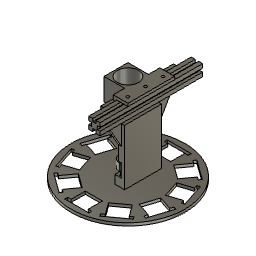
27.10_Derzhatel_motor_turel (Autodesk Fusion 360 design; units mm, degrees)
Autodesk Fusion 360 part; units mm, degrees
note: some values were not read from the file. Set by a fixed rule: which sketch regions a step uses.
sketch "Sketch1" plane through (0, 0, 0) normal (0, 0, 1) x (1, 0, 0)
  circle A0 centre (0, 0) radius 4
  dimension "d1" = 8
  constraint coincident A0.centre origin
  measures "d1" diameter of A0
sketch "Sketch2" plane through (0, 0, 0) normal (0, 0, 1) x (1, 0, 0)
  line L0 (-21, 21) -> (21, 21)
  line L1 (21, 21) -> (21, -21)
  line L2 (21, -21) -> (-21, -21)
  line L3 (-21, -21) -> (-21, 21)
  line L4 (-21, 21) -> (21, -21) construction
  circle A0 centre (0, 0) radius 4
  dimension "d4" = 42
  constraint horizontal L0
  constraint vertical L1
  constraint horizontal L2
  constraint vertical L3
  constraint equal L0 L3
  constraint midpoint A0.centre L4
  measures "d4" distance of L0.start L0.end
extrude "Extrude2" add sketch "Sketch2" along normal blind 8 makes body 1
sketch "Sketch3" plane through (0, 0, 8) normal (0, 0, 1) x (-1, 0, 0)
  circle A0 centre (0, 0) radius 4
  line L0 (21, 21) -> (-21, 21)
  line L1 (-21, 21) -> (-21, -21)
  line L2 (-21, -21) -> (21, -21)
  line L3 (21, -21) -> (21, 21)
  circle A1 centre (0, 0) radius 11.1
  line L4 (-10, 10) -> (10, 10)
  line L5 (10, 10) -> (10, -10)
  line L6 (10, -10) -> (-10, -10)
  line L7 (-10, -10) -> (-10, 10)
  line L8 (-10, 10) -> (10, -10) construction
  circle A2 centre (10, 10) radius 1.25
  circle A3 centre (10, -10) radius 1.25
  circle A4 centre (-10, 10) radius 1.25
  circle A5 centre (-10, -10) radius 1.25
  circle A6 centre (0, 0) radius 18.5
  dimension "d7" = 22.2
  dimension "d8" = 20
  dimension "d9" = 2.5
  dimension "d10" = 2.5
  dimension "d11" = 2.5
  dimension "d12" = 2.5
  dimension "d16" = 37
  constraint coincident A0.centre A1.centre
  constraint horizontal L4
  constraint vertical L5
  constraint horizontal L6
  constraint vertical L7
  constraint equal L4 L7
  constraint midpoint A0.centre L8
  constraint coincident L4.end L5.start
  constraint coincident L5.end L6.start
  constraint coincident L4.start L7.end
  constraint coincident L6.end L7.start
  measures "d7" diameter of A1
  measures "d8" distance of L4.start L4.end
  measures "d9" diameter of A2
  measures "d10" diameter of A3
  measures "d11" diameter of A4
  measures "d12" diameter of A5
  measures "d16" diameter of A6
extrude "Extrude3" cut sketch "Sketch3" against normal through all contours L4 L5 A2 | L4 L5 A2 | L5 L6 A3 | L5 L6 A3 | L4 L7 A4 | L4 L7 A4 | L6 L7 A5 | L6 L7 A5 bodies 1
extrude "Extrude4" cut sketch "Sketch3" against normal blind 2 contours A1 L5 | A1 L4 L5 L6 L7 | A1 L4 | A1 L6 | A1 L7 bodies 1
extrude "Extrude5" add sketch "Sketch3" along normal blind 31 contours L0 L1 L2 L3 bodies 1
sketch "Sketch4" plane through (21, 0, 0) normal (1, 0, 0) x (0, 1, 0)
  line L0 (-21, 0) -> (21, 0)
  line L1 (21, 0) -> (21, 39)
  line L2 (21, 39) -> (-21, 39)
  line L3 (-21, 39) -> (-21, 0)
  line L4 (-41, 39) -> (41, 39)
  line L5 (41, 39) -> (41, 14)
  line L6 (41, 14) -> (-41, 14)
  line L7 (-41, 14) -> (-41, 39)
  line L8 (-41, 39) -> (41, 39)
  line L9 (41, 39) -> (41, 34)
  line L10 (41, 34) -> (-41, 34)
  line L11 (-41, 34) -> (-41, 39)
  line L12 (21, 34) -> (41, 14) construction
  line L13 (41, 34) -> (21, 14) construction
  line L14 (41, 24.1296) -> (-41, 24.1296) construction
  circle A0 centre (31, 24) radius 2.5
  circle A1 centre (-31.4227, 24.1296) radius 2.5
  dimension "d19" = 25
  dimension "d20" = 20
  dimension "d21" = 20
  dimension "d24" = 5
  dimension "d27" = 5
  dimension "d28" = 5
  constraint horizontal L4
  constraint vertical L5
  constraint horizontal L6
  constraint vertical L7
  constraint horizontal L8
  constraint vertical L9
  constraint horizontal L10
  constraint vertical L11
  constraint coincident L1 L12.start
  constraint coincident L10 L12.start
  constraint coincident L6 L13.end
  constraint coincident L1 L13.end
  constraint coincident L5 L14.start
  constraint coincident L7 L14.end
  constraint perpendicular L7 L14
  constraint midpoint L13 A0.centre
  constraint coincident L14 A1.centre
  measures "d19" distance of L4.start L6.end
  measures "d20" distance of L3 L7
  measures "d21" distance of L1 L5
  measures "d24" distance of L4.start L10.end
  measures "d27" diameter of A0
  measures "d28" diameter of A1
extrude "Extrude6" add sketch "Sketch4" against normal blind 6 contours L3 L6 L7 L10 | L1 L5 L6 L10 | L3 L4 L7 L8 L10 L11 | L1 L4 L5 L8 L9 L10 | A0 | A1 bodies 1
extrude "Extrude7" add sketch "Sketch4" along normal blind 20 contours L3 L4 L7 L8 L10 L11 | L1 L2 L3 L4 L8 L10 | L1 L4 L5 L8 L9 L10 bodies 1
extrude "Extrude8" cut sketch "Sketch4" against normal through all contours A0 | A1 bodies 1
sketch "Sketch5" plane through (0, 0, 34) normal (0, 0, -1) x (1, 0, 0)
  line L0 (21, 41) -> (21, -41)
  line L1 (21, -41) -> (41, -41)
  line L2 (41, -41) -> (41, 41)
  line L3 (41, 41) -> (21, 41)
  line L4 (21, -41) -> (41, 41) construction
  line L5 (21, 41) -> (41, -41) construction
  line L6 (31, 41) -> (31, -41) construction
  circle A0 centre (31, 31.2813) radius 2.5
  circle A1 centre (31, 0) radius 2.5
  circle A2 centre (31, -30.6847) radius 2.5
  dimension "d30" = 5
  dimension "d31" = 5
  dimension "d32" = 5
  constraint coincident L0.end L1.start
  constraint coincident L2.end L3.start
  constraint coincident L0.start L3.end
  constraint coincident L1.end L2.start
  constraint midpoint L3 L6.start
  constraint perpendicular L3 L6
  constraint coincident L6 A0.centre
  constraint midpoint L5 A1.centre
  constraint coincident L6 A2.centre
  measures "d30" diameter of A0
  measures "d31" diameter of A1
  measures "d32" diameter of A2
extrude "Extrude9" cut sketch "Sketch5" against normal through all contours A0 | A1 | A2 bodies 1
ref_plane "WorkPlane1" through (0, 0, -2) normal (0, 0, -1) x (-1, 0, 0)
sketch "Sketch7" plane through (0, 0, -2) normal (0, 0, -1) x (1, 0, 0)
  circle A0 centre (0, 0) radius 4
  circle A1 centre (0, 0) radius 9.5
  dimension "d35" = 8
  dimension "d36" = 19
  constraint coincident A0.centre A1.centre
  measures "d35" diameter of A0
  measures "d36" diameter of A1
extrude "Extrude10" add sketch "Sketch7" along normal blind 19 separate body contours A0 | A1 makes body 2
sketch "Sketch10" plane through (0, 0, -21) normal (0, 0, -1) x (1, 0, 0)
  circle A0 centre (0, 0) radius 9.5
  circle A1 centre (0, 0) radius 4
extrude "Extrude13" add sketch "Sketch10" along normal blind 35 contours A1 bodies 2
sketch "Sketch11" plane through (0, 0, -56) normal (0, 0, -1) x (1, 0, 0)
  circle A0 centre (0, 0) radius 4
  line L0 (-6.5, -3.7528) -> (0, -7.5056)
  line L1 (0, -7.5056) -> (6.5, -3.7528)
  line L2 (6.5, -3.7528) -> (6.5, 3.7528)
  line L3 (6.5, 3.7528) -> (0, 7.5056)
  line L4 (0, 7.5056) -> (-6.5, 3.7528)
  line L5 (-6.5, 3.7528) -> (-6.5, -3.7528)
  dimension "d48" = 13
  constraint coincident A0.centre origin
  constraint vertical L5
  measures "d48" distance of L2 L5
extrude "Extrude14" add sketch "Sketch11" along normal blind 5 contours A0 | L0 L1 L2 L3 L4 L5 bodies 2
extrude "Extrude15" add sketch "Sketch7" against normal blind 10 contours A0 bodies 2
ref_plane "WorkPlane2" through (0, 0, -63) normal (0, 0, -1) x (-1, 0, 0)
sketch "Sketch12" plane through (0, 0, -63) normal (0, 0, -1) x (1, 0, 0)
  line L0 (-6.5, 3.7528) -> (-6.5, -3.7528)
  line L1 (-6.5, -3.7528) -> (0, -7.5056)
  line L2 (0, -7.5056) -> (6.5, -3.7528)
  line L3 (6.5, -3.7528) -> (6.5, 3.7528)
  line L4 (6.5, 3.7528) -> (0, 7.5056)
  line L5 (0, 7.5056) -> (-6.5, 3.7528)
extrude "Extrude16" add sketch "Sketch12" along normal blind 5 separate body makes body 3
sketch "Sketch13" plane through (0, 0, -68) normal (0, 0, -1) x (1, 0, 0)
  line L0 (0, 7.5056) -> (-6.5, 3.7528)
  line L1 (-6.5, 3.7528) -> (-6.5, -3.7528)
  line L2 (-6.5, -3.7528) -> (0, -7.5056)
  line L3 (0, -7.5056) -> (6.5, -3.7528)
  line L4 (6.5, -3.7528) -> (6.5, 3.7528)
  line L5 (6.5, 3.7528) -> (0, 7.5056)
  circle A0 centre (0, 0) radius 4
extrude "Extrude17" add sketch "Sketch13" along normal blind 45 contours A0 bodies 3
sketch "Sketch14" plane through (0, 0, -113) normal (0, 0, -1) x (1, 0, 0)
  circle A0 centre (0, 0) radius 4
  circle A1 centre (0, 0) radius 100
  line L0 (-21, -90) -> (21, -90)
  line L1 (21, -90) -> (21, -85)
  line L2 (21, -85) -> (15, -85)
  line L3 (15, -85) -> (15, -60)
  line L4 (15, -60) -> (-15, -60)
  line L5 (-15, -60) -> (-15, -85)
  line L6 (-15, -85) -> (-21, -85)
  line L7 (-21, -85) -> (-21, -90)
  line L8 (0, -60) -> (0, -90) construction
  line L9 (62.097, -59.9497) -> (47.4024, -39.7242)
  line L10 (47.4024, -39.7242) -> (23.1319, -57.3578)
  line L11 (23.1319, -57.3578) -> (37.8265, -77.5832)
  line L12 (37.8265, -77.5832) -> (32.9724, -81.1099)
  line L13 (32.9724, -81.1099) -> (35.9113, -85.155)
  line L14 (35.9113, -85.155) -> (69.89, -60.468)
  line L15 (69.89, -60.468) -> (66.9511, -56.423)
  line L16 (66.9511, -56.423) -> (62.097, -59.9497)
  line L17 (85.4751, -12.0006) -> (61.6986, -4.2752)
  line L18 (61.6986, -4.2752) -> (52.4281, -32.8069)
  line L19 (52.4281, -32.8069) -> (76.2045, -40.5323)
  line L20 (76.2045, -40.5323) -> (74.3504, -46.2386)
  line L21 (74.3504, -46.2386) -> (79.1057, -47.7837)
  line L22 (79.1057, -47.7837) -> (92.0844, -7.8393)
  line L23 (92.0844, -7.8393) -> (87.3292, -6.2943)
  line L24 (87.3292, -6.2943) -> (85.4751, -12.0006)
  line L25 (76.2045, 40.5323) -> (52.4281, 32.8069)
  line L26 (52.4281, 32.8069) -> (61.6986, 4.2752)
  line L27 (61.6986, 4.2752) -> (85.4751, 12.0006)
  line L28 (85.4751, 12.0006) -> (87.3292, 6.2943)
  line L29 (87.3292, 6.2943) -> (92.0844, 7.8393)
  line L30 (92.0844, 7.8393) -> (79.1057, 47.7837)
  line L31 (79.1057, 47.7837) -> (74.3504, 46.2386)
  line L32 (74.3504, 46.2386) -> (76.2045, 40.5323)
  line L33 (37.8265, 77.5832) -> (23.1319, 57.3578)
  line L34 (23.1319, 57.3578) -> (47.4024, 39.7242)
  line L35 (47.4024, 39.7242) -> (62.097, 59.9497)
  line L36 (62.097, 59.9497) -> (66.9511, 56.423)
  line L37 (66.9511, 56.423) -> (69.89, 60.468)
  line L38 (69.89, 60.468) -> (35.9113, 85.155)
  line L39 (35.9113, 85.155) -> (32.9724, 81.1099)
  line L40 (32.9724, 81.1099) -> (37.8265, 77.5832)
  line L41 (-15, 85) -> (-15, 60)
  line L42 (-15, 60) -> (15, 60)
  line L43 (15, 60) -> (15, 85)
  line L44 (15, 85) -> (21, 85)
  line L45 (21, 85) -> (21, 90)
  line L46 (21, 90) -> (-21, 90)
  line L47 (-21, 90) -> (-21, 85)
  line L48 (-21, 85) -> (-15, 85)
  line L49 (-62.097, 59.9497) -> (-47.4024, 39.7242)
  line L50 (-47.4024, 39.7242) -> (-23.1319, 57.3578)
  line L51 (-23.1319, 57.3578) -> (-37.8265, 77.5832)
  line L52 (-37.8265, 77.5832) -> (-32.9724, 81.1099)
  line L53 (-32.9724, 81.1099) -> (-35.9113, 85.155)
  line L54 (-35.9113, 85.155) -> (-69.89, 60.468)
  line L55 (-69.89, 60.468) -> (-66.9511, 56.423)
  line L56 (-66.9511, 56.423) -> (-62.097, 59.9497)
  line L57 (-85.4751, 12.0006) -> (-61.6986, 4.2752)
  line L58 (-61.6986, 4.2752) -> (-52.4281, 32.8069)
  line L59 (-52.4281, 32.8069) -> (-76.2045, 40.5323)
  line L60 (-76.2045, 40.5323) -> (-74.3504, 46.2386)
  line L61 (-74.3504, 46.2386) -> (-79.1057, 47.7837)
  line L62 (-79.1057, 47.7837) -> (-92.0844, 7.8393)
  line L63 (-92.0844, 7.8393) -> (-87.3292, 6.2943)
  line L64 (-87.3292, 6.2943) -> (-85.4751, 12.0006)
  line L65 (-76.2045, -40.5323) -> (-52.4281, -32.8069)
  line L66 (-52.4281, -32.8069) -> (-61.6986, -4.2752)
  line L67 (-61.6986, -4.2752) -> (-85.4751, -12.0006)
  line L68 (-85.4751, -12.0006) -> (-87.3292, -6.2943)
  line L69 (-87.3292, -6.2943) -> (-92.0844, -7.8393)
  line L70 (-92.0844, -7.8393) -> (-79.1057, -47.7837)
  line L71 (-79.1057, -47.7837) -> (-74.3504, -46.2386)
  line L72 (-74.3504, -46.2386) -> (-76.2045, -40.5323)
  line L73 (-37.8265, -77.5832) -> (-23.1319, -57.3578)
  line L74 (-23.1319, -57.3578) -> (-47.4024, -39.7242)
  line L75 (-47.4024, -39.7242) -> (-62.097, -59.9497)
  line L76 (-62.097, -59.9497) -> (-66.9511, -56.423)
  line L77 (-66.9511, -56.423) -> (-69.89, -60.468)
  line L78 (-69.89, -60.468) -> (-35.9113, -85.155)
  line L79 (-35.9113, -85.155) -> (-32.9724, -81.1099)
  line L80 (-32.9724, -81.1099) -> (-37.8265, -77.5832)
  dimension "d58" = 200
  dimension "d59" = 60
  dimension "d60" = 30
  dimension "d61" = 5
  dimension "d62" = 42
  dimension "d63" = 30
  dimension "d65" = 360
  constraint coincident A0.centre A1.centre
  constraint horizontal L0
  constraint perpendicular L0 L1
  constraint perpendicular L1 L2
  constraint perpendicular L2 L3
  constraint perpendicular L1 L4
  constraint perpendicular L4 L5
  constraint perpendicular L1 L6
  constraint perpendicular L0 L7
  constraint equal L2 L6
  constraint midpoint L4 L8.start
  constraint midpoint L0 L8.end
  constraint coincident A0.centre L8
  constraint equal L1 L7
  measures "d58" diameter of A1
  measures "d59" distance of A0.centre L4
  measures "d60" distance of L0 L4
  measures "d61" distance of L0.end L1.end
  measures "d62" distance of L0.start L0.end
  measures "d63" distance of L3.end L4.end
extrude "Extrude18" add sketch "Sketch14" along normal blind 5 contours A0 | A1 bodies 3
ref_plane "WorkPlane3" through (0, 0, -99) normal (0, 0, 1) x (-1, 0, 0)
sketch "Sketch15" plane through (0, 0, -99) normal (0, 0, 1) x (1, 0, 0)
  circle A0 centre (0, 0) radius 14.5
  line L0 (14.5, -27.5) -> (14.5, 27.5)
  line L1 (14.5, 27.5) -> (19.5, 27.5)
  line L2 (19.5, 27.5) -> (19.5, -27.5)
  line L3 (19.5, -27.5) -> (14.5, -27.5)
  circle A1 centre (0, 0) radius 4
  line L4 (19.5, 0) -> (14.5, 0) construction
  line L5 (0, -14.5) -> (14.5, -14.5)
  line L6 (0, 14.5) -> (14.5, 14.5)
  dimension "d69" = 29
  dimension "d74" = 8
  dimension "d77" = 5
  dimension "d78" = 55
  constraint coincident A0.centre A1.centre
  constraint concentric A0 A1
  constraint tangent A0 L0
  constraint vertical L0
  constraint vertical L2
  constraint horizontal L3
  constraint horizontal L1
  constraint midpoint L2 L4.start
  constraint midpoint L0 L4.end
  constraint coincident A0.centre L4
  constraint coincident A0 L5.start
  constraint coincident L0 L5.end
  constraint tangent A0 L5
  constraint coincident A0 L6.start
  constraint coincident L0 L6.end
  constraint tangent A0 L6
  constraint horizontal L5
  constraint horizontal L6
  measures "d69" diameter of A0
  measures "d74" diameter of A1
  measures "d77" distance of L0.start L2.end
  measures "d78" distance of L1.end L2.end
extrude "Extrude20" add sketch "Sketch15" along normal blind 13 bodies 3
sketch "Sketch16" plane through (0, 0, 0) normal (0, 1, 0) x (1, 0, 0)
  line L0 (21, -34) -> (41, -34)
  line L1 (21, -34) -> (21, -14)
  line L2 (21, -34) -> (41, -34)
  line L3 (21, -34) -> (21, -14)
  line L4 (21, -14) -> (41, -14)
  line L5 (41, -14) -> (41, -34)
  line L6 (31, -34) -> (31, -14) construction
  line L7 (41, -24) -> (21, -24) construction
  line L8 (21, -24) -> (21, -27)
  line L9 (21, -27) -> (26, -27)
  line L10 (26, -27) -> (26, -21)
  line L11 (26, -21) -> (21, -21)
  circle A0 centre (31, -24) radius 1.5 construction
  line L12 (28, -29) -> (28, -34)
  line L13 (34, -29) -> (28, -29)
  line L14 (34, -34) -> (34, -29)
  line L15 (36, -27) -> (41, -27)
  line L16 (36, -21) -> (36, -27)
  line L17 (41, -21) -> (36, -21)
  line L18 (34, -19) -> (34, -14)
  line L19 (28, -19) -> (34, -19)
  line L20 (28, -14) -> (28, -19)
  dimension "d81" = 3
  dimension "d82" = 6
  dimension "d83" = 5
  dimension "d84" = 3
  dimension "d86" = 360
  constraint coincident L0.start L1.start
  constraint coincident L0.end L2.end
  constraint coincident L1.end L3.end
  constraint perpendicular L3 L4
  constraint perpendicular L0 L5
  constraint midpoint L0 L6.start
  constraint midpoint L4 L6.end
  constraint midpoint L5 L7.start
  constraint midpoint L3 L7.end
  constraint perpendicular L7 L8
  constraint perpendicular L3 L9
  constraint perpendicular L7 L10
  constraint coincident L3 L11.end
  constraint perpendicular L3 L11
  constraint midpoint L7 A0.centre
  measures "d81" distance of L7.end L8.end
  measures "d82" distance of L9.end L10.end
  measures "d83" distance of L8.end L9.end
  measures "d84" diameter of A0
extrude "Extrude21" add sketch "Sketch16" along normal mid plane 180 separate body contours L0 L1 L2 L3 L4 L5 L9 L10 L11 L12 L13 L14 L15 L16 L17 L18 L19 L20 makes body 4
ref_plane "WorkPlane4" through (20.5, 0, -92.5) normal (1, 0, 0) x (0, 1, 0)
sketch "Sketch17" plane through (20.5, 0, -92.5) normal (1, 0, 0) x (0, 1, 0)
  line L0 (27.5, -6.5) -> (-27.5, -6.5)
  line L1 (-27.5, -6.5) -> (27.5, -6.5)
  line L2 (27.5, -6.5) -> (27.5, 6.5)
  line L3 (27.5, 6.5) -> (-27.5, 6.5)
  line L4 (-27.5, 6.5) -> (-27.5, -6.5)
  line L5 (-32.5, 6.5) -> (32.5, 6.5)
  line L6 (32.5, 6.5) -> (32.5, -11.5)
  line L7 (32.5, -11.5) -> (-32.5, -11.5)
  line L8 (-32.5, -11.5) -> (-32.5, 6.5)
  dimension "d88" = 5
  dimension "d89" = 5
  dimension "d90" = 5
  constraint horizontal L5
  constraint vertical L6
  constraint horizontal L7
  constraint vertical L8
  constraint collinear L3 L5
  measures "d88" distance of L2 L6
  measures "d89" distance of L4 L8
  measures "d90" distance of L0 L7
extrude "Extrude22" add sketch "Sketch17" along normal blind 6 separate body makes body 5
sketch "Sketch18" plane through (20.5, 0, 0) normal (-1, 0, 0) x (0, -1, 0)
  line L0 (-32.5, -104) -> (32.5, -104)
  line L1 (32.5, -104) -> (32.5, -86)
  line L2 (32.5, -86) -> (-32.5, -86)
  line L3 (-32.5, -86) -> (-32.5, -104)
  line L4 (27.5, -99) -> (14.5, -99)
  line L5 (-14.5, -99) -> (-27.5, -99)
  line L6 (-27.5, -99) -> (-14.5, -99)
  line L7 (-14.5, -99) -> (-14.5, -86)
  line L8 (-14.5, -86) -> (-27.5, -86)
  line L9 (-27.5, -86) -> (-27.5, -99)
  line L10 (14.5, -99) -> (27.5, -99)
  line L11 (27.5, -99) -> (27.5, -86)
  line L12 (27.5, -86) -> (14.5, -86)
  line L13 (14.5, -86) -> (14.5, -99)
  line L14 (32.5, -104) -> (21, -104)
  line L15 (21, -104) -> (21, -99)
  line L16 (21, -99) -> (32.5, -99)
  line L17 (32.5, -99) -> (32.5, -104)
  line L18 (-32.5, -104) -> (-21, -104)
  line L19 (-21, -104) -> (-21, -99)
  line L20 (-21, -99) -> (-32.5, -99)
  line L21 (-32.5, -99) -> (-32.5, -104)
  line L22 (-21, -104) -> (21, -104)
  line L23 (21, -104) -> (21, -99)
  line L24 (21, -99) -> (-21, -99)
  line L25 (-21, -99) -> (-21, -104)
  constraint horizontal L14
  constraint vertical L15
  constraint horizontal L16
  constraint vertical L17
  constraint midpoint L10 L15.end
  constraint coincident L0.end L1.start
  constraint horizontal L18
  constraint vertical L19
  constraint horizontal L20
  constraint vertical L21
  constraint midpoint L6 L19.end
  constraint coincident L0.start L3.end
  constraint horizontal L22
  constraint vertical L23
  constraint horizontal L24
  constraint vertical L25
extrude "Extrude23" add sketch "Sketch18" along normal blind 11 contours L0 L3 L5 L6 L18 L19 L20 L21 L25 | L0 L4 L5 L6 L10 L15 L19 L22 L23 L24 L25 | L0 L1 L4 L10 L14 L15 L16 L17 L23 bodies 5
sketch "Sketch19" plane through (0, 0, -99) normal (0, 0, 1) x (-1, 0, 0)
  line L0 (-9.5, -32.5) -> (-9.5, 32.5)
  line L1 (-9.5, 32.5) -> (-20.5, 32.5)
  line L2 (-20.5, 32.5) -> (-20.5, -32.5)
  line L3 (-20.5, -32.5) -> (-9.5, -32.5)
  circle A0 centre (0, 0) radius 4
  arc A1 (0, -14.5) -> (0, 14.5) centre (0, 0) ccw
  line L4 (0, 14.5) -> (-14.5, 14.5)
  line L5 (-14.5, 14.5) -> (-14.5, 27.5)
  line L6 (-14.5, 27.5) -> (-19.5, 27.5)
  line L7 (-19.5, 27.5) -> (-19.5, -27.5)
  line L8 (-19.5, -27.5) -> (-14.5, -27.5)
  line L9 (-14.5, -27.5) -> (-14.5, -14.5)
  line L10 (-14.5, -14.5) -> (0, -14.5)
  line L11 (-9.5, 32.5) -> (-14.5, 32.5)
  line L12 (-14.5, 32.5) -> (-14.5, 18.5)
  line L13 (-14.5, 18.5) -> (-9.5, 18.5)
  line L14 (-9.5, 18.5) -> (-9.5, 32.5)
  line L15 (-9.5, -32.5) -> (-14.5, -32.5)
  line L16 (-14.5, -32.5) -> (-14.5, -18.5)
  line L17 (-14.5, -18.5) -> (-9.5, -18.5)
  line L18 (-9.5, -18.5) -> (-9.5, -32.5)
  line L19 (-14.5, -32.5) -> (-20.5, -32.5)
  line L20 (-20.5, -32.5) -> (-20.5, -29.5)
  line L21 (-20.5, -29.5) -> (-14.5, -29.5)
  line L22 (-14.5, -29.5) -> (-14.5, -32.5)
  line L23 (-14.5, 32.5) -> (-20.5, 32.5)
  line L24 (-20.5, 32.5) -> (-20.5, 29.5)
  line L25 (-20.5, 29.5) -> (-14.5, 29.5)
  line L26 (-14.5, 29.5) -> (-14.5, 32.5)
  dimension "d95" = 14
  dimension "d99" = 2
  constraint horizontal L11
  constraint vertical L12
  constraint horizontal L13
  constraint vertical L14
  constraint coincident L5 L12.end
  constraint coincident L0.end L1.start
  constraint horizontal L15
  constraint vertical L16
  constraint horizontal L17
  constraint vertical L18
  constraint coincident L9 L16.end
  constraint coincident L0.start L3.end
  constraint equal L14 L18
  constraint horizontal L19
  constraint vertical L20
  constraint horizontal L21
  constraint vertical L22
  constraint coincident L2 L20.end
  constraint horizontal L23
  constraint vertical L24
  constraint horizontal L25
  constraint vertical L26
  constraint coincident L2 L24.end
  measures "d95" distance of L0.start L17.end
  measures "d99" distance of L8 L21
extrude "Extrude24" add sketch "Sketch19" along normal blind 10 contours L0 L3 L9 L15 L16 L17 L18 L22 | L2 L3 L16 L19 L20 L21 L22 | L0 L1 L5 L11 L12 L13 L14 L26 | L1 L2 L12 L23 L24 L25 L26 bodies 5
sketch "Sketch20" plane through (0, 0, -86) normal (0, 0, 1) x (-1, 0, 0)
  line L0 (-20.5, -32.5) -> (-20.5, 32.5)
  line L1 (-20.5, 32.5) -> (-26.5, 32.5)
  line L2 (-26.5, 32.5) -> (-26.5, -32.5)
  line L3 (-26.5, -32.5) -> (-20.5, -32.5)
extrude "Extrude25" add sketch "Sketch20" along normal blind 80 bodies 5
ref_plane "WorkPlane5" through (20.99, 0, 17.5) normal (-1, 0, 0) x (0, 0, 1)
sketch "Sketch21" plane through (20.99, 0, 17.5) normal (-1, 0, 0) x (0, 1, 0)
  circle A0 centre (-31.4227, -6.6296) radius 2.5
  line L0 (-21, 3.5) -> (-41, 3.5)
  line L1 (-41, 3.5) -> (-41, -21.5)
  line L2 (-41, -21.5) -> (-21, -21.5)
  line L3 (-21, -21.5) -> (-21, 3.5)
  circle A1 centre (31, -6.5) radius 2.5
  line L4 (41, -21.5) -> (41, 3.5)
  line L5 (41, 3.5) -> (21, 3.5)
  line L6 (21, 3.5) -> (21, -21.5)
  line L7 (21, -21.5) -> (41, -21.5)
  line L8 (-90, -16.5) -> (90, -16.5)
  line L9 (90, -16.5) -> (90, -9.5)
  line L10 (90, -9.5) -> (-90, -9.5)
  line L11 (-90, -9.5) -> (-90, -16.5)
  line L12 (-90, -3.5) -> (90, -3.5)
  line L13 (90, -3.5) -> (90, 3.5)
  line L14 (90, 3.5) -> (-90, 3.5)
  line L15 (-90, 3.5) -> (-90, -3.5)
  line L16 (-90, -9.5) -> (90, -9.5)
  line L17 (90, -9.5) -> (90, -3.5)
  line L18 (90, -3.5) -> (-90, -3.5)
  line L19 (-90, -3.5) -> (-90, -9.5)
  line L20 (-44, -16.5) -> (-64, -16.5)
  line L21 (-64, -16.5) -> (-64, 3.5)
  line L22 (-64, 3.5) -> (-44, 3.5)
  line L23 (-44, 3.5) -> (-44, -16.5)
  line L24 (44, -16.5) -> (64, -16.5)
  line L25 (64, -16.5) -> (64, 3.5)
  line L26 (64, 3.5) -> (44, 3.5)
  line L27 (44, 3.5) -> (44, -16.5)
  line L28 (32.5, 106.5) -> (29.5, 106.5)
  line L29 (29.5, 106.5) -> (29.5, 116.5)
  line L30 (29.5, 116.5) -> (-29.5, 116.5)
  line L31 (-29.5, 116.5) -> (-29.5, 106.5)
  line L32 (-29.5, 106.5) -> (-32.5, 106.5)
  line L33 (-32.5, 106.5) -> (-32.5, 23.5)
  line L34 (-32.5, 23.5) -> (32.5, 23.5)
  line L35 (32.5, 23.5) -> (32.5, 106.5)
  line L36 (-44, 3.5) -> (-32.5, 23.5)
  line L37 (-64, 3.5) -> (-32.5, 58.2826)
  line L38 (44, 3.5) -> (32.5, 23.5)
  line L39 (64, 3.5) -> (32.5, 58.2826)
  line L40 (31, -6.5) -> (-90, -6.5) construction
  line L41 (31, -6.5) -> (90, -6.5) construction
  line L42 (-54, -16.5) -> (-54, 3.5) construction
  line L43 (54, -16.5) -> (54, 3.5) construction
  circle A2 centre (-54, -6.5) radius 2.5
  circle A3 centre (54, -6.5) radius 2.5
  line L44 (-32.5, 23.5) -> (-27.5, 23.5)
  line L45 (-27.5, 23.5) -> (-27.5, 83.5)
  line L46 (-27.5, 83.5) -> (-32.5, 83.5)
  line L47 (-32.5, 83.5) -> (-32.5, 23.5)
  line L48 (32.5, 23.5) -> (27.5, 23.5)
  line L49 (27.5, 23.5) -> (27.5, 83.5)
  line L50 (27.5, 83.5) -> (32.5, 83.5)
  line L51 (32.5, 83.5) -> (32.5, 23.5)
  dimension "d103" = 20
  dimension "d104" = 3
  dimension "d105" = 3
  dimension "d106" = 5
  dimension "d107" = 5
  dimension "d108" = 5
  dimension "d109" = 5
  dimension "d110" = 60
  constraint horizontal L20
  constraint vertical L21
  constraint horizontal L22
  constraint vertical L23
  constraint coincident L14 L21.end
  constraint coincident L8 L20.start
  constraint horizontal L24
  constraint vertical L25
  constraint horizontal L26
  constraint vertical L27
  constraint coincident L14 L25.end
  constraint coincident L8 L24.start
  constraint equal L20 L24
  constraint coincident L33.end L34.start
  constraint coincident L33 L37.end
  constraint parallel L36 L37
  constraint coincident L34.end L35.start
  constraint coincident L35 L39.end
  constraint parallel L38 L39
  constraint coincident A1.centre L40.start
  constraint midpoint L19 L40.end
  constraint midpoint L17 L41.end
  constraint midpoint L20 L42.start
  constraint midpoint L22 L42.end
  constraint midpoint L24 L43.start
  constraint midpoint L26 L43.end
  constraint midpoint L42 A2.centre
  constraint midpoint L43 A3.centre
  constraint horizontal L44
  constraint vertical L45
  constraint horizontal L46
  constraint vertical L47
  constraint horizontal L48
  constraint vertical L49
  constraint horizontal L50
  constraint vertical L51
  constraint equal L45 L49
  measures "d103" distance of L24.start L24.end
  measures "d104" distance of L4 L27
  measures "d105" distance of L1 L23
  measures "d106" diameter of A2
  measures "d107" diameter of A3
  measures "d108" distance of L34.end L48.end
  measures "d109" distance of L33.end L44.end
  measures "d110" distance of L33.end L46.end
extrude "Extrude26" add sketch "Sketch21" along normal blind 5 contours L12 L14 L18 L21 L22 L23 | L14 L22 L33 L36 L37 L47 | L10 L12 L16 L18 L21 L23 | L33 L34 L44 L45 L46 L47 | L14 L26 L35 L38 L39 L51 | L12 L14 L18 L25 L26 L27 | L8 L10 L16 L20 L21 L23 | L10 L12 L16 L18 L25 L27 | L34 L35 L48 L49 L50 L51 | L8 L10 L16 L24 L25 L27 bodies 5
